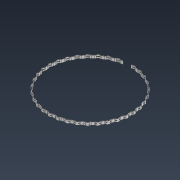
# Autodesk Inventor part: Pierścień zgarniający
Saved by Autodesk Inventor 2022 (Build 260153000, 153)
## iProperties
Created: 2023-04-17
Part Number: Pierścień zgarniający
Material: Generic
Document SubType Name: Modeling
Designer: wikto
Density: 1 g/cm^3
Appearance: Default
Author: wikto
Autodesk Inventor part; units mm, degrees
ref_plane "YZ Plane" through (0, 0, 0) normal (1, 0, 0) x (0, 1, 0)
ref_plane "XZ Plane" through (0, 0, 0) normal (0, 1, 0) x (-1, 0, 0)
sketch "Sketch2" plane through (0, 0, 0) normal (0, 1, 0) x (-1, 0, 0)
  circle A0 centre (0, 0) radius 41.5 construction
  circle A1 centre (0, 0) radius 42.5 construction
  arc A2 (0, -41.5) -> (-1.2758, -41.9598) centre (0, -43.5) ccw
  arc A3 (-4.011, -41.7871) -> (-1.2758, -41.9598) centre (-2.5516, -40.4195) ccw
  arc A4 (-4.011, -41.7871) -> (-5.2189, -41.1705) centre (-5.4704, -43.1547) ccw
  arc A5 (-7.4225, -40.8308) -> (-5.2189, -41.1705) centre (0, 0) ccw
  arc A6 (0, -42) -> (-0.9569, -42.3448) centre (0, -43.5) ccw
  arc A7 (-4.3758, -42.129) -> (-0.9569, -42.3448) centre (-2.5516, -40.4195) ccw
  arc A8 (-4.3758, -42.129) -> (-5.2817, -41.6666) centre (-5.4704, -43.1547) ccw
  arc A9 (-7.5119, -41.3228) -> (-5.2817, -41.6666) centre (0, 0) ccw
  arc A10 (-7.5119, -41.3228) -> (-8.515, -41.4909) centre (-7.7802, -42.7986) ccw
  arc A11 (-11.8402, -40.667) -> (-8.515, -41.4909) centre (-9.7397, -39.3114) ccw
  arc A12 (-7.4225, -40.8308) -> (-8.7599, -41.055) centre (-7.7802, -42.7986) ccw
  arc A13 (-11.4201, -40.3959) -> (-8.7599, -41.055) centre (-9.7397, -39.3114) ccw
  arc A14 (-11.8402, -40.667) -> (-12.6488, -40.0501) centre (-13.1006, -41.4804) ccw
  arc A15 (-11.4201, -40.3959) -> (-12.4982, -39.5733) centre (-13.1006, -41.4804) ccw
  arc A16 (-14.6055, -38.8449) -> (-12.4982, -39.5733) centre (0, 0) ccw
  arc A17 (-14.7815, -39.3129) -> (-12.6488, -40.0501) centre (0, 0) ccw
  arc A18 (-14.7815, -39.3129) -> (-15.7985, -39.2989) centre (-15.3094, -40.717) ccw
  arc A19 (-18.9228, -37.8936) -> (-15.7985, -39.2989) centre (-16.6137, -36.9356) ccw
  arc A20 (-14.6055, -38.8449) -> (-15.9615, -38.8263) centre (-15.3094, -40.717) ccw
  arc A21 (-18.461, -37.702) -> (-15.9615, -38.8263) centre (-16.6137, -36.9356) ccw
  arc A22 (-18.9228, -37.8936) -> (-19.608, -37.142) centre (-20.3083, -38.4685) ccw
  arc A23 (-18.461, -37.702) -> (-19.3746, -36.6998) centre (-20.3083, -38.4685) ccw
  arc A24 (-21.3176, -35.6063) -> (-19.3746, -36.6998) centre (0, 0) ccw
  arc A25 (-21.5745, -36.0353) -> (-19.608, -37.142) centre (0, 0) ccw
  arc A26 (-21.5745, -36.0353) -> (-22.5725, -35.8396) centre (-22.345, -37.3223) ccw
  arc A27 (-25.3951, -33.8982) -> (-22.5725, -35.8396) centre (-22.9519, -33.3686) ccw
  arc A28 (-21.3176, -35.6063) -> (-22.6484, -35.3454) centre (-22.345, -37.3223) ccw
  arc A29 (-24.9065, -33.7923) -> (-22.6484, -35.3454) centre (-22.9519, -33.3686) ccw
  arc A30 (-25.3951, -33.8982) -> (-25.9348, -33.0361) centre (-26.8611, -34.216) ccw
  arc A31 (-24.9065, -33.7923) -> (-25.6261, -32.6428) centre (-26.8611, -34.216) ccw
  arc A32 (-27.3422, -31.2194) -> (-25.6261, -32.6428) centre (0, 0) ccw
  arc A33 (-27.6716, -31.5956) -> (-25.9348, -33.0361) centre (0, 0) ccw
  arc A34 (-27.6716, -31.5956) -> (-28.6187, -31.2246) centre (-28.6599, -32.724) ccw
  arc A35 (-31.0485, -28.8096) -> (-28.6187, -31.2246) centre (-28.5499, -28.7255) ccw
  arc A36 (-27.3422, -31.2194) -> (-28.6049, -30.7247) centre (-28.6599, -32.724) ccw
  arc A37 (-30.5487, -28.7928) -> (-28.6049, -30.7247) centre (-28.5499, -28.7255) ccw
  arc A38 (-31.0485, -28.8096) -> (-31.4253, -27.8649) centre (-32.5476, -28.8601) ccw
  arc A39 (-30.5487, -28.7928) -> (-31.0512, -27.5332) centre (-32.5476, -28.8601) ccw
  arc A40 (-32.4851, -25.8258) -> (-31.0512, -27.5332) centre (0, 0) ccw
  arc A41 (-32.8765, -26.1369) -> (-31.4253, -27.8649) centre (0, 0) ccw
  arc A42 (-32.8765, -26.1369) -> (-33.7418, -25.6025) centre (-34.0506, -27.0704) ccw
  arc A43 (-35.7005, -22.7919) -> (-33.7418, -25.6025) centre (-33.2272, -23.1561) ccw
  arc A44 (-32.4851, -25.8258) -> (-33.6389, -25.1132) centre (-34.0506, -27.0704) ccw
  arc A45 (-35.2059, -22.8647) -> (-33.6389, -25.1132) centre (-33.2272, -23.1561) ccw
  arc A46 (-35.7005, -22.7919) -> (-35.9023, -21.795) centre (-37.1845, -22.5734) ccw
  arc A47 (-35.2059, -22.8647) -> (-35.4749, -21.5356) centre (-37.1845, -22.5734) ccw
  arc A48 (-36.5803, -19.5992) -> (-35.4749, -21.5356) centre (0, 0) ccw
  arc A49 (-37.021, -19.8354) -> (-35.9023, -21.795) centre (0, 0) ccw
  arc A50 (-37.021, -19.8354) -> (-37.7769, -19.1548) centre (-38.3432, -20.5438) ccw
  arc A51 (-39.2013, -16.0392) -> (-37.7769, -19.1548) centre (-36.833, -16.8398) ccw
  arc A52 (-36.5803, -19.5992) -> (-37.5881, -18.6918) centre (-38.3432, -20.5438) ccw
  arc A53 (-38.7277, -16.1993) -> (-37.5881, -18.6918) centre (-36.833, -16.8398) ccw
  arc A54 (-39.2013, -16.0392) -> (-39.2216, -15.0223) centre (-40.6223, -15.5588) ccw
  arc A55 (-38.7277, -16.1993) -> (-38.7546, -14.8435) centre (-40.6223, -15.5588) ccw
  arc A56 (-39.4959, -12.7407) -> (-38.7546, -14.8435) centre (0, 0) ccw
  arc A57 (-39.9717, -12.8942) -> (-39.2216, -15.0223) centre (0, 0) ccw
  arc A58 (-39.9717, -12.8942) -> (-40.5937, -12.0894) centre (-41.3993, -13.3547) ccw
  arc A59 (-41.4379, -8.7693) -> (-40.5937, -12.0894) centre (-39.251, -9.9806) ccw
  arc A60 (-39.4959, -12.7407) -> (-40.3251, -11.6676) centre (-41.3993, -13.3547) ccw
  arc A61 (-41.0005, -9.0115) -> (-40.3251, -11.6676) centre (-39.251, -9.9806) ccw
  arc A62 (-41.4379, -8.7693) -> (-41.2759, -7.7651) centre (-42.7501, -8.0425) ccw
  arc A63 (-41.0005, -9.0115) -> (-40.7846, -7.6727) centre (-42.7501, -8.0425) ccw
  arc A64 (-41.1378, -5.4712) -> (-40.7846, -7.6727) centre (0, 0) ccw
  arc A65 (-41.6334, -5.5372) -> (-41.2759, -7.7651) centre (0, 0) ccw
  arc A66 (-41.6334, -5.5372) -> (-42.1014, -4.6341) centre (-43.1203, -5.7349) ccw
  arc A67 (-42.3382, -1.2165) -> (-42.1014, -4.6341) centre (-40.4031, -2.7994) ccw
  arc A68 (-41.1378, -5.4712) -> (-41.7617, -4.2672) centre (-43.1203, -5.7349) ccw
  arc A69 (-41.9512, -1.5331) -> (-41.7617, -4.2672) centre (-40.4031, -2.7994) ccw
  arc A70 (-42.3382, -1.2165) -> (-41.9992, -0.2576) centre (-43.4992, -0.2668) ccw
  arc A71 (-41.9512, -1.5331) -> (-41.4992, -0.2545) centre (-43.4992, -0.2668) ccw
  arc A72 (-41.453, 1.9746) -> (-41.4992, -0.2545) centre (0, 0) ccw
  arc A73 (-41.9524, 1.9984) -> (-41.9992, -0.2576) centre (0, 0) ccw
  arc A74 (-41.9524, 1.9984) -> (-42.2513, 2.9706) centre (-43.4507, 2.0698) ccw
  arc A75 (-41.8731, 6.3755) -> (-42.2513, 2.9706) centre (-40.2523, 4.472) ccw
  arc A76 (-41.453, 1.9746) -> (-41.8515, 3.2709) centre (-43.4507, 2.0698) ccw
  arc A77 (-41.5489, 5.9948) -> (-41.8515, 3.2709) centre (-40.2523, 4.472) ccw
  arc A78 (-41.8731, 6.3755) -> (-41.3681, 7.2583) centre (-42.8455, 7.5176) ccw
  arc A79 (-41.5489, 5.9948) -> (-40.8756, 7.1719) centre (-42.8455, 7.5176) ccw
  arc A80 (-40.4314, 9.3569) -> (-40.8756, 7.1719) centre (0, 0) ccw
  arc A81 (-40.9185, 9.4696) -> (-41.3681, 7.2583) centre (0, 0) ccw
  arc A82 (-40.9185, 9.4696) -> (-41.0387, 10.4796) centre (-42.3799, 9.8078) ccw
  arc A83 (-40.0576, 13.7618) -> (-41.0387, 10.4796) centre (-38.8035, 11.5992) ccw
  arc A84 (-40.4314, 9.3569) -> (-40.5917, 10.7035) centre (-42.3799, 9.8078) ccw
  arc A85 (-39.8068, 13.3293) -> (-40.5917, 10.7035) centre (-38.8035, 11.5992) ccw
  arc A86 (-40.0576, 13.7618) -> (-39.4028, 14.5401) centre (-40.8101, 15.0594) ccw
  arc A87 (-39.8068, 13.3293) -> (-38.9338, 14.367) centre (-40.8101, 15.0594) ccw
  arc A88 (-38.106, 16.4373) -> (-38.9338, 14.367) centre (0, 0) ccw
  arc A89 (-38.5651, 16.6354) -> (-39.4028, 14.5401) centre (0, 0) ccw
  arc A90 (-38.5651, 16.6354) -> (-38.5027, 17.6505) centre (-39.9424, 17.2295) ccw
  arc A91 (-36.9503, 20.7044) -> (-38.5027, 17.6505) centre (-36.1032, 18.3523) ccw
  arc A92 (-38.106, 16.4373) -> (-38.0228, 17.7909) centre (-39.9424, 17.2295) ccw
  arc A93 (-36.7809, 20.234) -> (-38.0228, 17.7909) centre (-36.1032, 18.3523) ccw
  arc A94 (-36.9503, 20.7044) -> (-36.1669, 21.3531) centre (-37.4586, 22.1157) ccw
  arc A95 (-36.7809, 20.234) -> (-35.7364, 21.0989) centre (-37.4586, 22.1157) ccw
  arc A96 (-34.5516, 22.9877) -> (-35.7364, 21.0989) centre (0, 0) ccw
  arc A97 (-34.9679, 23.2646) -> (-36.1669, 21.3531) centre (0, 0) ccw
  arc A98 (-34.9679, 23.2646) -> (-34.725, 24.2523) centre (-36.2168, 24.0955) ccw
  arc A99 (-32.6515, 26.9793) -> (-34.725, 24.2523) centre (-32.2387, 24.5136) ccw
  arc A100 (-34.5516, 22.9877) -> (-34.2277, 24.3046) centre (-36.2168, 24.0955) ccw
  arc A101 (-32.5689, 26.4861) -> (-34.2277, 24.3046) centre (-32.2387, 24.5136) ccw
  arc A102 (-32.6515, 26.9793) -> (-31.7647, 27.4774) centre (-32.8991, 28.4587) ccw
  arc A103 (-32.5689, 26.4861) -> (-31.3865, 27.1503) centre (-32.8991, 28.4587) ccw
  arc A104 (-29.8831, 28.7967) -> (-31.3865, 27.1503) centre (0, 0) ccw
  arc A105 (-30.2431, 29.1437) -> (-31.7647, 27.4774) centre (0, 0) ccw
  arc A106 (-30.2431, 29.1437) -> (-29.8275, 30.072) centre (-31.3232, 30.1845) ccw
  arc A107 (-27.2996, 32.3841) -> (-29.8275, 30.072) centre (-27.3345, 29.8844) ccw
  arc A108 (-29.8831, 28.7967) -> (-29.3289, 30.0344) centre (-31.3232, 30.1845) ccw
  arc A109 (-27.3066, 31.8842) -> (-29.3289, 30.0344) centre (-27.3345, 29.8844) ccw
  arc A110 (-27.2996, 32.3841) -> (-26.338, 32.7156) centre (-27.2787, 33.884) ccw
  arc A111 (-27.3066, 31.8842) -> (-26.0245, 32.3261) centre (-27.2787, 33.884) ccw
  arc A112 (-24.2508, 33.6771) -> (-26.0245, 32.3261) centre (0, 0) ccw
  arc A113 (-24.543, 34.0829) -> (-26.338, 32.7156) centre (0, 0) ccw
  arc A114 (-24.543, 34.0829) -> (-23.968, 34.9218) centre (-25.4195, 35.3001) ccw
  arc A115 (-21.0674, 36.7446) -> (-23.968, 34.9218) centre (-21.5488, 34.2914) ccw
  arc A116 (-24.2508, 33.6771) -> (-23.4842, 34.7957) centre (-25.4195, 35.3001) ccw
  arc A117 (-21.1637, 36.2539) -> (-23.4842, 34.7957) centre (-21.5488, 34.2914) ccw
  arc A118 (-21.0674, 36.7446) -> (-20.062, 36.8987) centre (-20.7785, 38.2165) ccw
  arc A119 (-21.1637, 36.2539) -> (-19.8232, 36.4594) centre (-20.7785, 38.2165) ccw
  arc A120 (-17.8365, 37.4715) -> (-19.8232, 36.4594) centre (0, 0) ccw
  arc A121 (-18.0514, 37.9229) -> (-20.062, 36.8987) centre (0, 0) ccw
  arc A122 (-18.0514, 37.9229) -> (-17.3356, 38.6455) centre (-18.6961, 39.2773) ccw
  arc A123 (-14.1558, 39.9201) -> (-17.3356, 38.6455) centre (-15.0682, 37.5925) ccw
  arc A124 (-17.8365, 37.4715) -> (-16.8821, 38.4349) centre (-18.6961, 39.2773) ccw
  arc A125 (-14.3383, 39.4546) -> (-16.8821, 38.4349) centre (-15.0682, 37.5925) ccw
  arc A126 (-14.1558, 39.9201) -> (-13.1391, 39.8919) centre (-13.6083, 41.3166) ccw
  arc A127 (-14.3383, 39.4546) -> (-12.9826, 39.417) centre (-13.6083, 41.3166) ccw
  arc A128 (-10.847, 40.0574) -> (-12.9826, 39.417) centre (0, 0) ccw
  arc A129 (-10.9776, 40.54) -> (-13.1391, 39.8919) centre (0, 0) ccw
  arc A130 (-10.9776, 40.54) -> (-10.1442, 41.1229) centre (-11.3697, 41.9879) ccw
  arc A131 (-6.7876, 41.8082) -> (-10.1442, 41.1229) centre (-8.1016, 39.6814) ccw
  arc A132 (-10.847, 40.0574) -> (-9.7357, 40.8346) centre (-11.3697, 41.9879) ccw
  arc A133 (-7.0504, 41.3829) -> (-9.7357, 40.8346) centre (-8.1016, 39.6814) ccw
  arc A134 (-6.7876, 41.8082) -> (-5.7924, 41.5987) centre (-5.9992, 43.0843) ccw
  arc A135 (-7.0504, 41.3829) -> (-5.7234, 41.1034) centre (-5.9992, 43.0843) ccw
  arc A136 (-3.5076, 41.3515) -> (-5.7234, 41.1034) centre (0, 0) ccw
  arc A137 (-3.5499, 41.8497) -> (-5.7924, 41.5987) centre (0, 0) ccw
  arc A138 (-3.5499, 41.8497) -> (-2.6256, 42.2742) centre (-3.6767, 43.3443) ccw
  arc A139 (0.7994, 42.3481) -> (-2.6256, 42.2742) centre (-0.8738, 40.4906) ccw
  arc A140 (-3.5076, 41.3515) -> (-2.2752, 41.9175) centre (-3.6767, 43.3443) ccw
  arc A141 (0.4648, 41.9766) -> (-2.2752, 41.9175) centre (-0.8738, 40.4906) ccw
  arc A142 (0.7994, 42.3481) -> (1.7411, 41.9639) centre (1.8033, 43.4626) ccw
  arc A143 (0.4648, 41.9766) -> (1.7204, 41.4643) centre (1.8033, 43.4626) ccw
  arc A144 (3.9448, 41.3121) -> (1.7204, 41.4643) centre (0, 0) ccw
  arc A145 (3.9924, 41.8098) -> (1.7411, 41.9639) centre (0, 0) ccw
  arc A146 (3.9924, 41.8098) -> (4.9777, 42.0621) centre (4.1349, 43.303) ccw
  arc A147 (8.3606, 41.5223) -> (4.9777, 42.0621) centre (6.3822, 39.994) ccw
  arc A148 (3.9448, 41.3121) -> (5.2586, 41.6485) centre (4.1349, 43.303) ccw
  arc A149 (7.9649, 41.2166) -> (5.2586, 41.6485) centre (6.3822, 39.994) ccw
  arc A150 (8.3606, 41.5223) -> (9.2185, 40.9758) centre (9.5477, 42.4393) ccw
  arc A151 (7.9649, 41.2166) -> (9.1087, 40.488) centre (9.5477, 42.4393) ccw
  arc A152 (11.2701, 39.9404) -> (9.1087, 40.488) centre (0, 0) ccw
  arc A153 (11.4058, 40.4216) -> (9.2185, 40.9758) centre (0, 0) ccw
  arc A154 (11.4058, 40.4216) -> (12.4204, 40.4936) centre (11.8132, 41.8652) ccw
  arc A155 (15.6523, 39.3574) -> (12.4204, 40.4936) centre (13.4324, 38.2076) ccw
  arc A156 (11.2701, 39.9404) -> (12.6228, 40.0364) centre (11.8132, 41.8652) ccw
  arc A157 (15.2083, 39.1275) -> (12.6228, 40.0364) centre (13.4324, 38.2076) ccw
  arc A158 (15.6523, 39.3574) -> (16.3985, 38.6664) centre (16.9842, 40.0473) ccw
  arc A159 (15.2083, 39.1275) -> (16.2033, 38.2061) centre (16.9842, 40.0473) ccw
  arc A160 (18.2318, 37.2807) -> (16.2033, 38.2061) centre (0, 0) ccw
  arc A161 (18.4515, 37.7299) -> (16.3985, 38.6664) centre (0, 0) ccw
  arc A162 (18.4515, 37.7299) -> (19.4626, 37.6193) centre (19.1105, 39.0773) ccw
  arc A163 (22.4391, 35.9233) -> (19.4626, 37.6193) centre (20.0494, 35.1891) ccw
  arc A164 (18.2318, 37.2807) -> (19.5799, 37.1332) centre (19.1105, 39.0773) ccw
  arc A165 (21.9612, 35.7765) -> (19.5799, 37.1332) centre (20.0494, 35.1891) ccw
  arc A166 (22.4391, 35.9233) -> (23.0498, 35.1099) centre (23.873, 36.3639) ccw
  arc A167 (21.9612, 35.7765) -> (22.7754, 34.692) centre (23.873, 36.3639) ccw
  arc A168 (24.6057, 33.4187) -> (22.7754, 34.692) centre (0, 0) ccw
  arc A169 (24.9021, 33.8214) -> (23.0498, 35.1099) centre (0, 0) ccw
  arc A170 (24.9021, 33.8214) -> (25.8771, 33.5317) centre (25.7915, 35.0293) ccw
  arc A171 (28.5023, 31.3308) -> (25.8771, 33.5317) centre (26.0198, 31.0358) ccw
  arc A172 (24.6057, 33.4187) -> (25.9057, 33.0325) centre (25.7915, 35.0293) ccw
  arc A173 (28.0058, 31.2718) -> (25.9057, 33.0325) centre (26.0198, 31.0358) ccw
  arc A174 (28.5023, 31.3308) -> (28.9577, 30.4213) centre (29.9919, 31.5077) ccw
  arc A175 (28.0058, 31.2718) -> (28.6129, 30.0591) centre (29.9919, 31.5077) ccw
  arc A176 (30.186, 28.479) -> (28.6129, 30.0591) centre (0, 0) ccw
  arc A177 (30.5497, 28.8221) -> (28.9577, 30.4213) centre (0, 0) ccw
  arc A178 (30.5497, 28.8221) -> (31.4571, 28.3628) centre (31.6408, 29.8515) ccw
  arc A179 (33.6464, 25.7278) -> (31.4571, 28.3628) centre (31.1511, 25.8816) ccw
  arc A180 (30.186, 28.479) -> (31.3959, 27.8666) centre (31.6408, 29.8515) ccw
  arc A181 (33.1473, 25.7586) -> (31.3959, 27.8666) centre (31.1511, 25.8816) ccw
  arc A182 (33.6464, 25.7278) -> (33.9317, 24.7515) centre (35.1436, 25.6355) ccw
  arc A183 (33.1473, 25.7586) -> (33.5278, 24.4569) centre (35.1436, 25.6355) ccw
  arc A184 (34.7929, 22.6209) -> (33.5278, 24.4569) centre (0, 0) ccw
  arc A185 (35.2121, 22.8935) -> (33.9317, 24.7515) centre (0, 0) ccw
  arc A186 (35.2121, 22.8935) -> (36.0227, 22.2792) centre (36.4696, 23.7111) ccw
  arc A187 (37.7054, 19.2952) -> (36.0227, 22.2792) centre (35.2779, 19.8928) ccw
  arc A188 (34.7929, 22.6209) -> (35.8738, 21.8019) centre (36.4696, 23.7111) ccw
  arc A189 (37.2199, 19.4147) -> (35.8738, 21.8019) centre (35.2779, 19.8928) ccw
  arc A190 (37.7054, 19.2952) -> (37.8115, 18.2836) centre (39.1619, 18.9366) ccw
  arc A191 (37.2199, 19.4147) -> (37.3614, 18.0659) centre (39.1619, 18.9366) ccw
  arc A192 (38.2777, 16.0333) -> (37.3614, 18.0659) centre (0, 0) ccw
  arc A193 (38.7389, 16.2265) -> (37.8115, 18.2836) centre (0, 0) ccw
  arc A194 (38.7389, 16.2265) -> (39.4266, 15.4772) centre (40.1224, 16.806) ccw
  arc A195 (40.5484, 12.2403) -> (39.4266, 15.4772) centre (38.2669, 13.2624) ccw
  arc A196 (38.2777, 16.0333) -> (39.1947, 15.0342) centre (40.1224, 16.806) ccw
  arc A197 (40.0921, 12.4447) -> (39.1947, 15.0342) centre (38.2669, 13.2624) ccw
  arc A198 (40.5484, 12.2403) -> (40.4719, 11.226) centre (41.9173, 11.627) ccw
  arc A199 (40.0921, 12.4447) -> (39.9901, 11.0924) centre (41.9173, 11.627) ccw
  arc A200 (40.5281, 8.9287) -> (39.9901, 11.0924) centre (0, 0) ccw
  arc A201 (41.0164, 9.0362) -> (40.4719, 11.226) centre (0, 0) ccw
  arc A202 (41.0164, 9.0362) -> (41.559, 8.176) centre (42.4813, 9.359) ccw
  arc A203 (42.0838, 4.7906) -> (41.559, 8.176) centre (40.0219, 6.2043) ccw
  arc A204 (40.5281, 8.9287) -> (41.2516, 7.7817) centre (42.4813, 9.359) ccw
  arc A205 (41.6715, 5.0734) -> (41.2516, 7.7817) centre (40.0219, 6.2043) ccw
  arc A206 (42.0838, 4.7906) -> (41.8272, 3.8065) centre (43.321, 3.9424) ccw
  arc A207 (41.6715, 5.0734) -> (41.3292, 3.7611) centre (43.321, 3.9424) ccw
  arc A208 (41.4716, 1.5361) -> (41.3292, 3.7611) centre (0, 0) ccw
  arc A209 (41.9712, 1.5546) -> (41.8272, 3.8065) centre (0, 0) ccw
  arc A210 (41.9712, 1.5546) -> (42.3512, 0.6111) centre (43.4702, 1.6101) ccw
  arc A211 (42.2621, -2.8135) -> (42.3512, 0.6111) centre (40.4863, -1.0538) ccw
  arc A212 (41.4716, 1.5361) -> (41.9782, 0.2781) centre (43.4702, 1.6101) ccw
  arc A213 (41.9069, -2.4616) -> (41.9782, 0.2781) centre (40.4863, -1.0538) ccw
  arc A214 (42.2621, -2.8135) -> (41.8335, -3.7359) centre (43.3276, -3.8693) ccw
  arc A215 (41.9069, -2.4616) -> (41.3355, -3.6914) centre (43.3276, -3.8693) ccw
  arc A216 (41.0776, -5.9061) -> (41.3355, -3.6914) centre (0, 0) ccw
  arc A217 (41.5725, -5.9772) -> (41.8335, -3.7359) centre (0, 0) ccw
  arc A218 (41.5725, -5.9772) -> (41.7776, -6.9734) centre (43.0572, -6.1907) ccw
  arc A219 (41.0774, -10.3269) -> (41.7776, -6.9734) centre (39.645, -8.2779) ccw
  arc A220 (41.0776, -5.9061) -> (41.3511, -7.2343) centre (43.0572, -6.1907) ccw
  arc A221 (40.7909, -9.9171) -> (41.3511, -7.2343) centre (39.645, -8.2779) ccw
  arc A222 (41.0774, -10.3269) -> (40.4908, -11.1577) centre (41.9369, -11.5562) ccw
  arc A223 (40.7909, -9.9171) -> (40.0088, -11.0249) centre (41.9369, -11.5562) ccw
  arc A224 (39.3589, -13.1577) -> (40.0088, -11.0249) centre (0, 0) ccw
  arc A225 (39.8331, -13.3163) -> (40.4908, -11.1577) centre (0, 0) ccw
  arc A226 (39.8331, -13.3163) -> (39.8568, -14.3331) centre (41.2557, -13.7918) ccw
  arc A227 (38.5681, -17.5072) -> (39.8568, -14.3331) centre (37.5252, -15.2351) ccw
  arc A228 (39.3589, -13.1577) -> (39.3905, -14.5135) centre (41.2557, -13.7918) ccw
  arc A229 (38.3595, -17.0528) -> (39.3905, -14.5135) centre (37.5252, -15.2351) ccw
  arc A230 (38.5681, -17.5072) -> (37.8423, -18.2198) centre (39.1938, -18.8705) ccw
  arc A231 (38.3595, -17.0528) -> (37.3918, -18.0029) centre (39.1938, -18.8705) ccw
  arc A232 (36.371, -19.9851) -> (37.3918, -18.0029) centre (0, 0) ccw
  arc A233 (36.8092, -20.2259) -> (37.8423, -18.2198) centre (0, 0) ccw
  arc A234 (36.8092, -20.2259) -> (36.6506, -21.2305) centre (38.1238, -20.9482) ccw
  arc A235 (34.8149, -24.123) -> (36.6506, -21.2305) centre (34.1953, -21.701) ccw
  arc A236 (36.371, -19.9851) -> (36.1595, -21.3246) centre (38.1238, -20.9482) ccw
  arc A237 (34.691, -23.6386) -> (36.1595, -21.3246) centre (34.1953, -21.701) ccw
  arc A238 (34.8149, -24.123) -> (33.9734, -24.6943) centre (35.1868, -25.5762) ccw
  arc A239 (34.691, -23.6386) -> (33.569, -24.4003) centre (35.1868, -25.5762) ccw
  arc A240 (32.2101, -26.1679) -> (33.569, -24.4003) centre (0, 0) ccw
  arc A241 (32.5982, -26.4832) -> (33.9734, -24.6943) centre (0, 0) ccw
  arc A242 (32.5982, -26.4832) -> (32.2624, -27.4433) centre (33.7624, -27.429) ccw
  arc A243 (29.9391, -29.9608) -> (32.2624, -27.4433) centre (29.7626, -27.4671) ccw
  arc A244 (32.2101, -26.1679) -> (31.7625, -27.4481) centre (33.7624, -27.429) ccw
  arc A245 (29.9038, -29.4621) -> (31.7625, -27.4481) centre (29.7626, -27.4671) ccw
  arc A246 (29.9391, -29.9608) -> (29.009, -30.3724) centre (30.045, -31.4571) ccw
  arc A247 (29.9038, -29.4621) -> (28.6636, -30.0108) centre (30.045, -31.4571) ccw
  arc A248 (27.0105, -31.5069) -> (28.6636, -30.0108) centre (0, 0) ccw
  arc A249 (27.3359, -31.8865) -> (29.009, -30.3724) centre (0, 0) ccw
  arc A250 (27.3359, -31.8865) -> (26.8339, -32.7711) centre (28.3122, -33.0253) ccw
  arc A251 (24.0977, -34.8325) -> (26.8339, -32.7711) centre (24.37, -32.3473) ccw
  arc A252 (27.0105, -31.5069) -> (26.3411, -32.6863) centre (28.3122, -33.0253) ccw
  arc A253 (24.1522, -34.3354) -> (26.3411, -32.6863) centre (24.37, -32.3473) ccw
  arc A254 (24.0977, -34.8325) -> (23.109, -35.071) centre (23.9343, -36.3235) ccw
  arc A255 (24.1522, -34.3354) -> (22.8339, -34.6535) centre (23.9343, -36.3235) ccw
  arc A256 (20.9398, -35.8298) -> (22.8339, -34.6535) centre (0, 0) ccw
  arc A257 (21.1921, -36.2615) -> (23.109, -35.071) centre (0, 0) ccw
  arc A258 (21.1921, -36.2615) -> (20.5399, -37.042) centre (21.9489, -37.5565) ccw
  arc A259 (17.4792, -38.5808) -> (20.5399, -37.042) centre (18.1916, -36.1845) ccw
  arc A260 (20.9398, -35.8298) -> (20.0703, -36.8705) centre (21.9489, -37.5565) ccw
  arc A261 (17.6217, -38.1015) -> (20.0703, -36.8705) centre (18.1916, -36.1845) ccw
  arc A262 (17.4792, -38.5808) -> (16.4638, -38.6386) centre (17.0517, -40.0186) ccw
  arc A263 (17.6217, -38.1015) -> (16.2678, -38.1787) centre (17.0517, -40.0186) ccw
  arc A264 (14.1938, -38.9972) -> (16.2678, -38.1787) centre (0, 0) ccw
  arc A265 (14.3648, -39.4671) -> (16.4638, -38.6386) centre (0, 0) ccw
  arc A266 (14.3648, -39.4671) -> (13.5836, -40.1184) centre (14.8779, -40.8766) ccw
  arc A267 (10.297, -41.0849) -> (13.5836, -40.1184) centre (11.4266, -38.8546) ccw
  arc A268 (14.1938, -38.9972) -> (13.1522, -39.8656) centre (14.8779, -40.8766) ccw
  arc A269 (10.5229, -40.6389) -> (13.1522, -39.8656) centre (11.4266, -38.8546) ccw
  arc A270 (10.297, -41.0849) -> (9.2876, -40.9602) centre (9.6193, -42.4231) ccw
  arc A271 (10.5229, -40.6389) -> (9.177, -40.4726) centre (9.6193, -42.4231) ccw
  arc A272 (6.9901, -40.9071) -> (9.177, -40.4726) centre (0, 0) ccw
  arc A273 (7.0744, -41.3999) -> (9.2876, -40.9602) centre (0, 0) ccw
  line L0 (0, -42) -> (0, -41.5)
  line L1 (7.0744, -41.3999) -> (6.9901, -40.9071)
  point P0 (-7.4225, -40.8308)
  point P1 (-14.6055, -38.8449)
  point P2 (-21.3176, -35.6063)
  point P3 (-27.3422, -31.2194)
  point P4 (-32.4851, -25.8258)
  point P5 (-36.5803, -19.5992)
  point P6 (-39.4959, -12.7407)
  point P7 (-41.1378, -5.4712)
  point P8 (-41.453, 1.9746)
  point P9 (-40.4314, 9.3569)
  point P10 (-38.106, 16.4373)
  point P11 (-34.5516, 22.9877)
  point P12 (-29.8831, 28.7967)
  point P13 (-24.2508, 33.6771)
  point P14 (-17.8365, 37.4715)
  point P15 (-10.847, 40.0574)
  point P16 (-3.5076, 41.3515)
  point P17 (3.9448, 41.3121)
  point P18 (11.2701, 39.9404)
  point P19 (18.2318, 37.2807)
  point P20 (24.6057, 33.4187)
  point P21 (30.186, 28.479)
  point P22 (34.7929, 22.6209)
  point P23 (38.2777, 16.0333)
  point P24 (40.5281, 8.9287)
  point P25 (41.4716, 1.5361)
  point P26 (41.0776, -5.9061)
  point P27 (39.3589, -13.1577)
  point P28 (36.371, -19.9851)
  point P29 (32.2101, -26.1679)
  point P30 (27.0105, -31.5069)
  point P31 (20.9398, -35.8298)
  point P32 (14.1938, -38.9972)
  point P33 (14.3648, -39.4671)
  point P34 (21.1921, -36.2615)
  point P35 (27.3359, -31.8865)
  point P36 (32.5982, -26.4832)
  point P37 (36.8092, -20.2259)
  point P38 (39.8331, -13.3163)
  point P39 (41.5725, -5.9772)
  point P40 (41.9712, 1.5546)
  point P41 (41.0164, 9.0362)
  point P42 (38.7389, 16.2265)
  point P43 (35.2121, 22.8935)
  point P44 (30.5497, 28.8221)
  point P45 (24.9021, 33.8214)
  point P46 (18.4515, 37.7299)
  point P47 (11.4058, 40.4216)
  point P48 (3.9924, 41.8098)
  point P49 (-3.5499, 41.8497)
  point P50 (-10.9776, 40.54)
  point P51 (-18.0514, 37.9229)
  point P52 (-24.543, 34.0829)
  point P53 (-30.2431, 29.1437)
  point P54 (-34.9679, 23.2646)
  point P55 (-38.5651, 16.6354)
  point P56 (-40.9185, 9.4696)
  point P57 (-41.9524, 1.9984)
  point P58 (-41.6334, -5.5372)
  point P59 (-39.9717, -12.8942)
  point P60 (-37.021, -19.8354)
  point P61 (-32.8765, -26.1369)
  point P62 (-27.6716, -31.5956)
  point P63 (-21.5745, -36.0353)
  point P64 (-14.7815, -39.3129)
  point P65 (-7.5119, -41.3228)
  dimension "d14" = 83
  dimension "d15" = 85
  dimension "d17" = 2
  dimension "d19" = 0.5
  dimension "d22" = 340
  constraints: 547 point on circle, 274 centre point, 5 coincident, 5 tangent, 4 end point, 2 equal radius, 1 concentric, 1 vertical, 1 vertical alignment, 729 other
  measures "d14" diameter of A0
  measures "d15" diameter of A1
  measures "d17" radius of A3
  measures "d19" radial gap between concentric circles of A2 A6
extrude "Extrusion1" add sketch "Sketch2" along normal blind 3
ref_plane "Work Plane1" through (0, 1.5, 0) normal (0, 1, 0) x (1, 0, 0)
sketch "Sketch5" plane through (0, 1.5, 0) normal (0, 1, 0) x (1, 0, 0)
  arc A0 (0, 41.5) -> (1.2758, 41.9598) centre (0, 43.5) ccw projected
  circle A1 centre (0, 0) radius 41.5 construction
  circle A2 centre (0, 0) radius 43 construction
  arc A3 (4.3758, 42.129) -> (0.9569, 42.3448) centre (2.5516, 40.4195) ccw projected
  circle A4 centre (0, 0) radius 42.5 construction
  dimension "d26" = 0.5
  constraints: 3 coincident, 2 centre point, 1 tangent, 1 vertical alignment, 2 other
  measures "d26" radial gap between concentric circles of A4 A2
sketch "Sketch6" plane through (0, 0, -42) normal (-1, 0, 0) x (0, 0, 1)
  line L0 (42, -0.6) -> (42, 3.6) projected
  line L1 (85, 1.5) -> (-1, 1.5) construction
  line L2 (83.5, 1.5) -> (0.5, 1.5) construction
  circle A0 centre (-0.6, 1.5) radius 0.25
  circle A1 centre (-0.35, 1.5) radius 0.25
  line L3 (0, 0) -> (0, 3) projected
  line L4 (-0.6, 1.25) -> (-0.35, 1.25)
  line L5 (-0.6, 1.75) -> (-0.35, 1.75)
  point P0 (42, 0)
  dimension "d30" = 0.1
  dimension "d31" = 0.5
  dimension "d32" = 0.4
  constraints: 4 end point, 4 point on circle, 2 centre point, 2 horizontal, 2 point on line, 2 vertical alignment, 1 equal radius
  measures "d30" distance edge to line of A1 L3
  measures "d31" diameter of A0
  measures "d32" distance of A0.centre L1.end
revolve "Revolution1" cut sketch "Sketch6" angle 360 about axis through (0, -10, 0) along (0, 1, 0)
body "Solid1"
